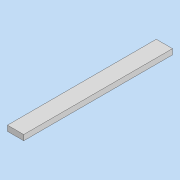
# Autodesk Inventor part: bodyBotPlate
Saved by Autodesk Inventor 2021 (Build 250183000, 183)
## iProperties
Created: 2021-02-01
Part Number: bodyBotPlate
Material: Generic
Document SubType Name: Modeling
Designer: garre
Density: 1 g/cm^3
Appearance: Default
Author: garre
Autodesk Inventor part; units mm, degrees
ref_plane "YZ Plane" through (0, 0, 0) normal (1, 0, 0) x (0, 1, 0)
ref_plane "XZ Plane" through (0, 0, 0) normal (0, 1, 0) x (-1, 0, 0)
ref_plane "XY Plane" through (0, 0, 0) normal (0, 0, 1) x (1, 0, 0)
sketch "Sketch1" plane through (0, 0, 0) normal (0, 1, 0) x (-1, 0, 0)
  line L0 (0, 0) -> (76.2, 0)
  line L1 (76.2, 0) -> (76.2, -698.5)
  line L2 (76.2, -698.5) -> (0, -698.5)
  line L3 (0, -698.5) -> (0, 0)
  dimension "d0" = 698.5
  dimension "d1" = 76.2
  constraints: 8 end point, 2 parallel, 1 horizontal, 1 perpendicular
  measures "d0" distance of L0.end L1.end
  measures "d1" distance of L0.start L0.end
extrude "Extrusion1" add sketch "Sketch1" along normal blind 25.4
equation "\"d0\" = botPlateLength"
equation "\"d1\" = botPlateWidth"
equation "\"d2\" = woodThickness"
equation "\"botPlateLength\" = 698.5"
equation "\"botPlateWidth\" = 76.2"
equation "\"woodThickness\" = 25.4"
body "Solid1"
